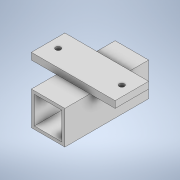
# Autodesk Inventor part: Motor Mount
Saved by Autodesk Inventor 2021 (Build 250183000, 183)
## iProperties
Created: 2020-04-12
Part Number: Motor Mount
Material: Generic
Document SubType Name: Modeling
Designer: chutsu
Density: 1 g/cm^3
Appearance: Default
Author: chutsu
Autodesk Inventor part; units mm, degrees
ref_plane "YZ Plane" through (0, 0, 0) normal (1, 0, 0) x (0, 1, 0)
ref_plane "XZ Plane" through (0, 0, 0) normal (0, 1, 0) x (-1, 0, 0)
ref_plane "XY Plane" through (0, 0, 0) normal (0, 0, 1) x (1, 0, 0)
sketch "Sketch1" plane through (0, 0, 0) normal (0, 1, 0) x (-1, 0, 0)
  line L0 (5, -12.5) -> (-5, -12.5)
  line L1 (-5, -12.5) -> (-5, 12.5)
  line L2 (-5, 12.5) -> (5, 12.5)
  line L3 (5, 12.5) -> (5, -12.5)
  line L4 (5, 0) -> (-5, 0)
  line L5 (0, -12.5) -> (0, 12.5)
  point P0 (0, 0)
  dimension "d1" = 10
  dimension "d2" = 25
  constraints: 12 end point, 6 midpoint, 2 parallel, 1 horizontal, 1 perpendicular
  measures "d1" distance between parallel lines of L1 L3
  measures "d2" distance between parallel lines of L2 L0
extrude "Extrusion1" add sketch "Sketch1" along normal blind 10
sketch "Sketch2" plane through (-5, 0, 12.5) normal (0, 0, 1) x (1, 0, 0)
  line L0 (10, 0) -> (10, 10) projected
  line L1 (0, 0) -> (10, 0) projected
  line L2 (0, 0) -> (0, 10) projected
  line L3 (0, 10) -> (10, 10) projected
  line L4 (5, 10) -> (5, 0)
  line L5 (0.9, 9.1) -> (9.1, 9.1)
  line L6 (9.1, 9.1) -> (9.1, 0.9)
  line L7 (9.1, 0.9) -> (0.9, 0.9)
  line L8 (0.9, 0.9) -> (0.9, 9.1)
  line L9 (5, 9.1) -> (5, 0.9)
  line L10 (0, 5) -> (10, 5)
  line L11 (0.9, 5) -> (9.1, 5)
  line L12 (5, 9.1) -> (5, 0.9)
  point P0 (5, 5)
  point P1 (5, 5)
  dimension "d9" = 8.2
  dimension "d10" = 8.2
  constraints: 18 end point, 11 midpoint, 3 perpendicular, 2 parallel, 1 horizontal
  measures "d9" distance of L5.start L5.end
  measures "d10" distance between parallel lines of L7 L5
extrude "Extrusion2" cut sketch "Sketch2" against normal through all contours L10 L4 L5 L6 | L6 L7 L4 L10 | L7 L8 L10 L4 | L10 L8 L5 L4
sketch "Sketch5" plane through (0, 10, 0) normal (0, 1, 0) x (1, 0, 0)
  line L0 (-12.5, 5) -> (12.5, 5)
  line L1 (12.5, 5) -> (12.5, -5)
  line L2 (12.5, -5) -> (-12.5, -5)
  line L3 (-12.5, -5) -> (-12.5, 5)
  line L4 (-12.5, 0) -> (12.5, 0)
  line L5 (0, 5) -> (0, -5)
  point P0 (0, 0)
  dimension "d32" = 25
  dimension "d33" = 10
  constraints: 12 end point, 6 midpoint, 2 parallel, 1 horizontal, 1 perpendicular
  measures "d32" distance between parallel lines of L1 L3
  measures "d33" distance between parallel lines of L2 L0
extrude "Extrusion4" add sketch "Sketch5" along normal blind 2
sketch "Sketch7" plane through (0, 12, 0) normal (0, 1, 0) x (1, 0, 0)
  line L0 (-12.5, 5) -> (-12.5, -5) projected
  line L1 (-12.5, 0) -> (12.5, 0)
  line L2 (12.5, -5) -> (12.5, 5) projected
  point P0 (0, 0)
  point P1 (-9.5, 0)
  point P2 (9.5, 0)
  dimension "d53" = 19
  dimension "d54" = 9.5
  constraints: 2 end point, 2 midpoint, 2 point on line
  measures "d53" distance of point (9.5, 0) point (-9.5, 0)
  measures "d54" distance of point (0, 0) point (9.5, 0)
hole "Hole3" at (9.5, 12, 0) at (-9.5, 12, 0) direction (0, -1, 0) diameter 1.55 end through all
body "Solid1"
